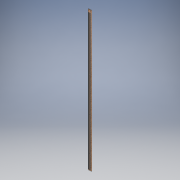
# Autodesk Inventor part: træhåndfang
Saved by Autodesk Inventor 2018 (Build 220112000, 112)
## iProperties
Created: 2019-09-28
Part Number: træhåndfang
Material: Wood (Birch)
Document SubType Name: Modeling
Designer: loppen
Density: 0.55 g/cm^3
Appearance: Birch - Natural Polished
Mass: 11829.5 g
Surface Area: 12525.9 cm^2
Volume: 21508.1 cm^3
Author: loppen
Autodesk Inventor part; units mm, degrees
ref_plane "YZ Plane" through (0, 0, 0) normal (1, 0, 0) x (0, 1, 0)
ref_plane "XZ Plane" through (0, 0, 0) normal (0, 1, 0) x (-1, 0, 0)
ref_plane "XY Plane" through (0, 0, 0) normal (0, 0, 1) x (1, 0, 0)
sketch "Sketch1" plane through (0, 0, 0) normal (0, 0, 1) x (1, 0, 0)
  line L0 (-56, 0) -> (56, 0) projected
  line L1 (40, -20) -> (40, 20)
  line L2 (40, 20) -> (-40, 20)
  line L3 (-40, 20) -> (-40, -20)
  line L4 (-40, -20) -> (40, -20)
  point P0 (0, 0)
  dimension "d8" = 80
  dimension "d9" = 40
  dimension "d11" = 40
  constraints: 8 end point, 1 horizontal, 1 parallel, 1 perpendicular, 1 other
  measures "d8" distance of L1.end L2.end
  measures "d9" distance of L1.start L1.end
  measures "d11" distance from line of point (0, 0) L3
extrude "Extrusion1" add sketch "Sketch1" along normal mid plane 5000
sketch "Sketch2" plane through (40, -20, -2500) normal (0, -1, 0) x (1, 0, 0)
  line L0 (0, 5000) -> (0, 0) projected
  line L1 (-80, 5000) -> (0, 5000) projected
  line L2 (-80, 0) -> (-80, 5000) projected
  line L3 (0, 0) -> (-80, 0) projected
  line L4 (-40, -1000) -> (-40, 6000) projected
  line L5 (-12.5, 52.621) -> (-67.5, 52.621)
  line L6 (-70.5, 55.621) -> (-70.5, 4894.172)
  line L7 (-67.5, 4897.172) -> (-12.5, 4897.172)
  line L8 (-9.5, 4894.172) -> (-9.5, 55.621)
  arc A0 (-70.5, 55.621) -> (-67.5, 52.621) centre (-67.5, 55.621) ccw
  arc A1 (-12.5, 52.621) -> (-9.5, 55.621) centre (-12.5, 55.621) ccw
  arc A2 (-67.5, 4897.172) -> (-70.5, 4894.172) centre (-67.5, 4894.172) ccw
  arc A3 (-9.5, 4894.172) -> (-12.5, 4897.172) centre (-12.5, 4894.172) ccw
  point P0 (-40, 2500)
  dimension "d12" = 61
  dimension "d13" = 4844.551
  dimension "d14" = 3
  dimension "d29" = 52.621
  constraints: 8 end point, 8 point on circle, 8 tangent, 4 centre point, 3 equal radius, 2 parallel, 1 horizontal, 1 perpendicular, 1 other
  measures "d12" distance between parallel lines of L8 L6
  measures "d13" distance between parallel lines of L7 L5
  measures "d14" radius of A0
  measures "d29" distance between parallel lines of L3 L5
extrude "Extrusion2" cut sketch "Sketch2" against normal blind 5 contours L7 A3 L8 A1 L5 L4 | L4 L5 A0 L6 A2 L7
sketch "Sketch3" plane through (40, -15, -2500) normal (0, -1, 0) x (1, 0, 0)
  line L0 (-70.5, 55.621) -> (-70.5, 4894.172) projected
  arc A0 (-70.5, 55.621) -> (-67.5, 52.621) centre (-67.5, 55.621) ccw projected
  line L1 (-12.5, 52.621) -> (-67.5, 52.621) projected
  arc A1 (-12.5, 52.621) -> (-9.5, 55.621) centre (-12.5, 55.621) ccw projected
  line L2 (-9.5, 4894.172) -> (-9.5, 55.621) projected
  arc A2 (-9.5, 4894.172) -> (-12.5, 4897.172) centre (-12.5, 4894.172) ccw projected
  line L3 (-67.5, 4897.172) -> (-12.5, 4897.172) projected
  arc A3 (-67.5, 4897.172) -> (-70.5, 4894.172) centre (-67.5, 4894.172) ccw projected
  line L4 (-40, 4890.172) -> (-40, 59.621) construction
  line L5 (-46, 4890.172) -> (-46, 59.621)
  line L6 (-34, 59.621) -> (-34, 4890.172)
  arc A4 (-34, 4890.172) -> (-46, 4890.172) centre (-40, 4890.172) ccw
  arc A5 (-46, 59.621) -> (-34, 59.621) centre (-40, 59.621) ccw
  line L7 (-40, -1000) -> (-40, 6000) projected
  point P0 (-40, 2500)
  point P1 (-40, 2474.8965)
  dimension "d19" = 12
  dimension "d22" = 1
  dimension "d23" = 1
  constraints: 8 end point, 4 point on circle, 4 tangent, 2 centre point, 1 collinear, 1 midpoint, 1 parallel, 1 vertical
  measures "d19" diameter of A5
  measures "d22" distance edge to line of A5 L1
  measures "d23" distance edge to line of A4 L3
extrude "Extrusion3" cut sketch "Sketch3" against normal blind 16 contours L7 A4 L6 A5 | A5 L5 A4 L7
sketch "Sketch4" plane through (40, 1, -2500) normal (0, -1, 0) x (1, 0, 0)
  line L0 (-46, 59.621) -> (-46, 4890.172) projected
  arc A0 (-46, 59.621) -> (-34, 59.621) centre (-40, 59.621) ccw projected
  line L1 (-34, 4890.172) -> (-34, 59.621) projected
  arc A1 (-34, 4890.172) -> (-46, 4890.172) centre (-40, 4890.172) ccw projected
  line L2 (-40, -1000) -> (-40, 6000) projected
  line L3 (-40, 4891.172) -> (-40, 58.621) construction
  line L4 (-45, 4891.172) -> (-45, 58.621)
  line L5 (-35, 58.621) -> (-35, 4891.172)
  arc A2 (-35, 4891.172) -> (-45, 4891.172) centre (-40, 4891.172) ccw
  arc A3 (-45, 58.621) -> (-35, 58.621) centre (-40, 58.621) ccw
  point P0 (-40, 2500)
  point P1 (-40, 2474.8965)
  dimension "d24" = 10
  dimension "d25" = 0
  dimension "d26" = 0
  constraints: 8 end point, 4 point on circle, 4 tangent, 2 centre point, 2 point on line, 1 midpoint, 1 parallel
  measures "d24" diameter of A3
  measures "d25" horizontal distance between centres of A0 A3
  measures "d26" horizontal distance between centres of A1 A2
extrude "Extrusion4" cut sketch "Sketch4" against normal blind 7 contours A3 L4 A2 L2 | L2 A2 L5 A3
sketch "Sketch5" plane through (40, 20, 2500) normal (1, 0, 0) x (0, 0, -1)
  line L0 (0, 0) -> (5000, 0) projected
  line L1 (0, -40) -> (0, 0) projected
  line L2 (0, -40) -> (5000, -40) projected
  line L3 (5000, 0) -> (5000, -40) projected
  line L4 (5000, 0) -> (5000, -40) projected
  line L5 (5000, 0) -> (4972.7139, -40)
  line L6 (0, -40) -> (5000, -40) projected
  point P0 (2500, -20)
  dimension "d30" = 34.3
  constraints: 2 end point, 1 point on line
  measures "d30" angle of L3 L5
extrude "endeafskær top" cut sketch "Sketch5" against normal through all contours L3 L2 L5
sketch "Sketch6" plane through (40, 20, 2500) normal (1, 0, 0) x (0, 0, -1)
  line L0 (4972.7139, -40) -> (5000, 0) projected
  line L1 (0, 0) -> (5000, 0) projected
  line L2 (0, -40) -> (0, 0) projected
  line L3 (0, -40) -> (4972.7139, -40) projected
  line L4 (0, -40) -> (0, 0) projected
  line L5 (0, -40) -> (27.2861, 0)
  point P0 (2500, -20)
  dimension "d33" = 34.3
  constraints: 2 end point, 1 point on line
  measures "d33" angle of L2 L5
extrude "endeafskær bund" cut sketch "Sketch6" against normal through all contours L2 L1 L5
fillet "Fillet2" [suppressed]
fillet "Fillet3" [suppressed]
fillet "Fillet4" [suppressed]
fillet "Fillet5" [suppressed]
sketch "Sketch7" plane through (40, -15, -2500) normal (0, -1, 0) x (1, 0, 0)
  ellipse E0 centre (-40, 549.6501) end of major axis (-40, 574.4656) minor radius 20.5 projected
  ellipse E1 centre (-40, 1760.3552) end of major axis (-40, 1785.1707) minor radius 20.5 projected
  ellipse E2 centre (-40, 2971.3032) end of major axis (-40, 2996.1187) minor radius 20.5 projected
  line L0 (-93.9939, 549.6501) -> (45.3161, 549.6501) construction
  line L1 (-103.3896, 1760.3552) -> (51.928, 1760.3552) construction
  line L2 (-132.8398, 2971.3032) -> (53.2138, 2971.3032) construction
  line L3 (-45, 58.621) -> (-45, 4891.172) construction
  arc A0 (-45, 58.621) -> (-35, 58.621) centre (-40, 58.621) ccw construction
  line L4 (-35, 4891.172) -> (-35, 58.621) construction
  arc A1 (-35, 4891.172) -> (-45, 4891.172) centre (-40, 4891.172) ccw construction
  circle A2 centre (-45, 549.6501) radius 6
  circle A3 centre (-35, 549.6501) radius 6
  circle A4 centre (-35, 1760.3552) radius 6
  circle A5 centre (-45, 1760.3552) radius 6
  circle A6 centre (-45, 2971.3032) radius 6
  circle A7 centre (-35, 2971.3032) radius 6
  point P0 (-40, 2500)
  dimension "d38" = 12
  dimension "d39" = 12
  dimension "d40" = 12
  dimension "d41" = 12
  dimension "d42" = 12
  dimension "d43" = 12
  constraints: 12 point on line, 6 centre point, 6 end point, 3 horizontal, 3 other
  measures "d38" diameter of A2
  measures "d39" diameter of A3
  measures "d40" diameter of A4
  measures "d41" diameter of A5
  measures "d42" diameter of A6
  measures "d43" diameter of A7
extrude "Extrusion7" cut sketch "Sketch7" against normal up to surface (23 mm away) contours A2 A3 | A2 A3 | A3 A2 | A4 A5 | A5 A4 | A4 A5 | A6 A7 | A6 A7 | A7 A6
equation "\"d11\" = 0.5 * d8"
equation "\"d30\" = trappevinkel"
equation "\"d33\" = trappevinkel"
equation "\"d39\" = d38"
equation "\"d40\" = d38"
equation "\"d41\" = d38"
equation "\"d42\" = d38"
equation "\"d43\" = d38"
equation "\"pladetykkelse\" = 3"
equation "\"trappevinkel\" = 34.3deg"
equation "\"trappestifter_dia\" = 25"
equation "\"trappestifter_huldia\" = 25.8"
equation "\"trappestifter_skraa_huldia\" = 26.6"
equation "\"trappestifter_laengde\" = 228"
equation "\"perforeringsbredde\" = 6"
equation "\"perforeringshullaengde\" = 62.8"
equation "\"perforeringshullaengde_top\" = 61"
equation "\"perforeringshullaengde_bund\" = 61.6"
equation "\"perforeringsoffset\" = 8"
equation "\"perforeringsoffset_top\" = 8"
equation "\"perforeringsoffset_bund\" = 8"
equation "\"laskehul_dia\" = 13"
equation "\"balusterhul_udvidelse\" = 1"
equation "\"trinbredde\" = 1884"
body "Solid1"
